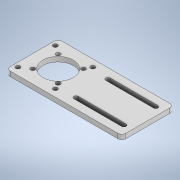
# Autodesk Inventor part: NEMA23_FaceMount
Saved by Autodesk Inventor 2021 (Build 250183000, 183)
## iProperties
Created: 2021-10-05
Part Number: NEMA23_FaceMount
Material: Generic
Document SubType Name: Modeling
Designer: Jorian Brusind
Density: 1 g/cm^3
Appearance: Default
Author: Jorian Brusind
Autodesk Inventor part; units mm, degrees
ref_plane "YZ Plane" through (0, 0, 0) normal (1, 0, 0) x (0, 1, 0)
ref_plane "XZ Plane" through (0, 0, 0) normal (0, 1, 0) x (-1, 0, 0)
ref_plane "XY Plane" through (0, 0, 0) normal (0, 0, 1) x (1, 0, 0)
sketch "Sketch1" plane through (0, 0, 0) normal (0, 1, 0) x (-1, 0, 0)
  line L0 (0, 0) -> (65, 0)
  line L1 (65, 0) -> (65, -65)
  line L2 (65, -65) -> (0, -65)
  line L3 (0, -65) -> (0, 0)
  line L4 (0, 0) -> (-80, 0)
  line L5 (-80, 0) -> (-80, -65)
  line L6 (-80, -65) -> (0, -65)
  line L7 (0, -65) -> (0, 0)
  circle A0 centre (59.49, -9) radius 2.75
  circle A1 centre (59.49, -56) radius 2.75
  circle A2 centre (12.49, -9) radius 2.75
  circle A3 centre (12.49, -56) radius 2.75
  line L8 (-40, 0) -> (-40, -12.5)
  line L9 (-40, -12.5) -> (-40, -52.5)
  line L10 (-70, -12.5) -> (-10, -12.5) construction
  line L11 (-70, -15.25) -> (-10, -15.25)
  line L12 (-10, -9.75) -> (-70, -9.75)
  arc A4 (-70, -9.75) -> (-70, -15.25) centre (-70, -12.5) ccw
  arc A5 (-10, -15.25) -> (-10, -9.75) centre (-10, -12.5) ccw
  line L13 (-70, -52.5) -> (-10, -52.5) construction
  line L14 (-70, -55.25) -> (-10, -55.25)
  line L15 (-10, -49.75) -> (-70, -49.75)
  arc A6 (-70, -49.75) -> (-70, -55.25) centre (-70, -52.5) ccw
  arc A7 (-10, -55.25) -> (-10, -49.75) centre (-10, -52.5) ccw
  line L16 (-40, -52.5) -> (20, -52.5) construction
  circle A8 centre (32.5, -32.5) radius 22.5
  line L17 (32.5, -32.5) -> (48.4099, -16.5901)
  line L18 (32.5, -32.5) -> (55, -32.5) construction
  circle A9 centre (48.4099, -16.5901) radius 2.75
  circle A10 centre (16.5901, -16.5901) radius 2.75
  circle A11 centre (16.5901, -48.4099) radius 2.75
  circle A12 centre (48.4099, -48.4099) radius 2.75
  circle A13 centre (32.5, -32.5) radius 19.1
  dimension "d31" = 45
  dimension "d0" = 65
  dimension "d1" = 65
  dimension "d2" = 80
  dimension "d3" = 65
  dimension "d4" = 5.5
  dimension "d5" = 5.51
  dimension "d6" = 9
  dimension "d9" = 47
  dimension "d12" = 47
  dimension "d15" = 12.5
  dimension "d16" = 40
  dimension "d17" = 30
  dimension "d18" = 5.5
  dimension "d19" = 30
  dimension "d20" = 0
  dimension "d21" = 5.5
  dimension "d32" = 32.5
  dimension "d33" = 32.5
  dimension "d34" = 45
  dimension "d35" = 5.5
  dimension "d38" = 360
  dimension "d40" = 38.2
  constraints: 42 end point, 13 centre point, 8 point on circle, 8 tangent, 7 parallel, 6 horizontal, 3 midpoint, 3 vertical, 2 coincident, 2 equal length, 2 perpendicular, 18 other
  measures "d0" distance of L1.end L2.end
  measures "d1" distance of L0.end L1.end
  measures "d2" distance of L6.end L5.end
  measures "d3" distance of L5.end L4.end
  measures "d4" diameter of A0
  measures "d5" distance from line of L1 A0.centre
  measures "d6" distance from line of L0 A0.centre
  measures "d9" distance of A0.centre A1.centre
  measures "d12" distance of A0.centre A2.centre
  measures "d15" distance of L8.start L8.end
  measures "d16" distance of L8.end L9.end
  measures "d17" distance of L8.end L10.end
  measures "d18" diameter of A5
  measures "d19" distance of L9.end L13.end
  measures "d20" distance between parallel lines of L13 L16
  measures "d21" diameter of A7
  measures "d32" distance from line of L0 L17.start
  measures "d33" distance from line of L1 L17.start
  measures "d34" angle of L18 L17
  measures "d35" diameter of A9
  measures "d40" diameter of A13
extrude "Extrusion3" add sketch "Sketch1" along normal blind 6 contours L0 L1 L2 L3 | L3 L6 L5 L4 | A8 A12 A11 A10 A9
fillet "Fillet3" radius 5 4 edges at (-65, 3, 0) (-65, 3, -65) (80, 3, -65) (80, 3, 0)
body "Solid3"
